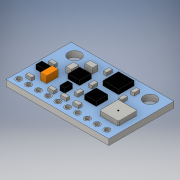
# Autodesk Inventor part: GY81
Saved by Autodesk Inventor 2016 (Build 200138000, 138)
## iProperties
Created: 2015-11-27
Part Number: GY81
Material: Generic
Document SubType Name: Modeling
Designer: Spooner
Density: 1 g/cm^3
Appearance: Default
Author: Spooner
Autodesk Inventor part; units mm, degrees
ref_plane "YZ Plane" through (0, 0, 0) normal (1, 0, 0) x (0, 1, 0)
ref_plane "XZ Plane" through (0, 0, 0) normal (0, 1, 0) x (-1, 0, 0)
ref_plane "XY Plane" through (0, 0, 0) normal (0, 0, 1) x (1, 0, 0)
sketch "Sketch1" plane through (0, 0, 0) normal (0, 1, 0) x (-1, 0, 0)
  line L0 (0, 0) -> (-26.67, 0)
  line L1 (-26.67, 0) -> (-26.67, -16.891)
  line L2 (-26.67, -16.891) -> (0, -16.891)
  line L3 (0, -16.891) -> (0, 0)
  circle A0 centre (-3.5369, -14.2431) radius 1.632
  circle A1 centre (-23.133, -14.2431) radius 1.632
  dimension "d0" = 16.891
  dimension "d1" = 26.67
  dimension "d2" = 3.2639
  dimension "d3" = 1.016
  dimension "d4" = 1.905
  dimension "d5" = 1.905
  constraints: 8 end point, 2 centre point, 2 parallel, 1 equal radius, 1 horizontal, 1 horizontal alignment, 1 perpendicular
  measures "d0" distance of L2.end L0.start
  measures "d1" distance of L1.end L2.end
  measures "d2" diameter of A0
  measures "d3" distance edge to line of A0 L2
  measures "d4" distance edge to line of A0 L3
  measures "d5" distance edge to line of A1 L1
extrude "Board" add sketch "Sketch1" along normal blind 1.524
sketch "Sketch2" plane through (0, 1.524, 0) normal (0, 1, 0) x (1, 0, 0)
  line L0 (20.1803, 4.0513) -> (25.0698, 4.0513)
  line L1 (25.0698, 4.0513) -> (25.0698, 8.9408)
  line L2 (25.0698, 8.9408) -> (20.1803, 8.9408)
  line L3 (20.1803, 8.9408) -> (20.1803, 4.0513)
  line L4 (26.67, 0) -> (26.67, 16.891) projected
  line L5 (26.67, 16.891) -> (0, 16.891) projected
  point P0 (0, 0)
  dimension "d8" = 4.8895
  dimension "d9" = 1.6002
  dimension "d10" = 7.9502
  constraints: 8 end point, 2 parallel, 2 perpendicular, 1 horizontal
  measures "d8" distance of L0.start L0.end
  measures "d9" distance between parallel lines of L4 L1
  measures "d10" distance between parallel lines of L2 L5
extrude "BMP085 Barometer" add sketch "Sketch2" along normal blind 1.1176
fillet "BMP085 Barometer Fillets" radius 0.254 4 edges at (25.0698, 2.0828, -4.0513) (20.1803, 2.0828, -4.0513) (20.1803, 2.0828, -8.9408) (25.0698, 2.0828, -8.9408)
sketch "Sketch3" plane through (0, 2.6416, 0) normal (0, 1, 0) x (1, 0, 0)
  circle A0 centre (22.6251, 6.4961) radius 0.1905
  line L0 (24.8158, 8.9408) -> (20.4343, 8.9408) projected
  line L1 (20.1803, 8.6868) -> (20.1803, 4.3053) projected
  point P0 (0, 0)
  point P1 (22.6251, 8.9408)
  point P2 (20.1803, 6.4961)
  dimension "d14" = 0.381
  constraints: 2 midpoint, 1 centre point, 1 horizontal alignment, 1 vertical alignment
  measures "d14" diameter of A0
extrude "BMP085 Barometer Hole" cut sketch "Sketch3" against normal blind 0.0254
sketch "Sketch4" plane through (0, 1.524, 0) normal (0, 1, 0) x (1, 0, 0)
  line L0 (13.97, 15.24) -> (18.034, 15.24)
  line L1 (18.034, 15.24) -> (18.034, 11.176)
  line L2 (18.034, 11.176) -> (13.97, 11.176)
  line L3 (13.97, 11.176) -> (13.97, 15.24)
  line L4 (14.7193, 8.6868) -> (17.7673, 8.6868)
  line L5 (17.7673, 8.6868) -> (17.7673, 5.6388)
  line L6 (17.7673, 5.6388) -> (14.7193, 5.6388)
  line L7 (14.7193, 5.6388) -> (14.7193, 8.6868)
  line L8 (7.874, 11.2141) -> (10.922, 11.2141)
  line L9 (10.922, 11.2141) -> (10.922, 8.1661)
  line L10 (10.922, 8.1661) -> (7.874, 8.1661)
  line L11 (7.874, 8.1661) -> (7.874, 11.2141)
  line L12 (9.4361, 6.5532) -> (10.7061, 6.5532)
  line L13 (10.7061, 6.5532) -> (10.7061, 4.5212)
  line L14 (10.7061, 4.5212) -> (9.4361, 4.5212)
  line L15 (9.4361, 4.5212) -> (9.4361, 6.5532)
  line L16 (1.6129, 7.6581) -> (4.1529, 7.6581)
  line L17 (4.1529, 7.6581) -> (4.1529, 6.1341)
  line L18 (4.1529, 6.1341) -> (1.6129, 6.1341)
  line L19 (1.6129, 6.1341) -> (1.6129, 7.6581)
  line L20 (26.67, 16.891) -> (0, 16.891) projected
  line L21 (26.67, 0) -> (26.67, 16.891) projected
  line L22 (20.1803, 4.3053) -> (20.1803, 8.6868) projected
  line L23 (0, 16.891) -> (0, 0) projected
  dimension "d17" = 4.064
  dimension "d18" = 3.048
  dimension "d19" = 1.27
  dimension "d20" = 2.032
  dimension "d21" = 1.524
  dimension "d22" = 2.54
  dimension "d23" = 1.651
  dimension "d24" = 8.636
  dimension "d25" = 2.413
  dimension "d26" = 2.4892
  dimension "d27" = 3.048
  dimension "d28" = 5.6769
  dimension "d29" = 4.0132
  dimension "d30" = 1.6129
  dimension "d31" = 1.6129
  dimension "d32" = 9.2329
  constraints: 40 end point, 10 parallel, 5 horizontal, 5 perpendicular, 4 equal length
  measures "d17" distance of L0.start L0.end
  measures "d18" distance of L4.start L4.end
  measures "d19" distance of L12.start L12.end
  measures "d20" distance of L14.end L12.start
  measures "d21" distance of L18.end L16.start
  measures "d22" distance of L16.start L16.end
  measures "d23" distance between parallel lines of L20 L0
  measures "d24" distance between parallel lines of L21 L1
  measures "d25" distance between parallel lines of L22 L5
  measures "d26" distance between parallel lines of L2 L4
  measures "d27" distance between parallel lines of L3 L9
  measures "d28" distance between parallel lines of L20 L8
  measures "d29" distance between parallel lines of L7 L13
  measures "d30" distance between parallel lines of L10 L12
  measures "d31" distance between parallel lines of L23 L19
  measures "d32" distance between parallel lines of L16 L20
extrude "Extrusion4" add sketch "Sketch4" along normal blind 1.1684
sketch "Sketch5" plane through (0, 1.524, 0) normal (0, 1, 0) x (1, 0, 0)
  line L0 (4.572, 7.366) -> (6.1849, 7.366)
  line L1 (6.1849, 7.366) -> (6.1849, 4.318)
  line L2 (6.1849, 4.318) -> (4.572, 4.318)
  line L3 (4.572, 4.318) -> (4.572, 7.366)
  line L4 (0, 0) -> (26.67, 0) projected
  line L5 (0, 16.891) -> (0, 0) projected
  dimension "d35" = 1.6129
  dimension "d36" = 3.048
  dimension "d74" = 4.318
  dimension "d75" = 4.572
  constraints: 8 end point, 2 parallel, 1 horizontal, 1 perpendicular
  measures "d35" distance of L1.end L2.end
  measures "d36" distance of L2.end L0.start
  measures "d74" distance between parallel lines of L4 L2
  measures "d75" distance between parallel lines of L5 L3
extrude "Extrusion5" add sketch "Sketch5" along normal blind 1.7399
sketch "Sketch6" plane through (0, 1.524, 0) normal (0, 1, 0) x (1, 0, 0)
  line L0 (8.0137, 13.843) -> (9.9949, 13.843)
  line L1 (9.9949, 13.843) -> (9.9949, 12.446)
  line L2 (9.9949, 12.446) -> (8.0137, 12.446)
  line L3 (8.0137, 12.446) -> (8.0137, 13.843)
  line L4 (0, 16.891) -> (0, 0) projected
  line L5 (6.2357, 11.2649) -> (7.6327, 11.2649)
  line L6 (7.6327, 11.2649) -> (7.6327, 9.2837)
  line L7 (7.6327, 9.2837) -> (6.2357, 9.2837)
  line L8 (6.2357, 9.2837) -> (6.2357, 11.2649)
  line L9 (26.67, 16.891) -> (0, 16.891) projected
  dimension "d39" = 1.9812
  dimension "d41" = 8.0137
  dimension "d42" = 1.397
  dimension "d43" = 6.2357
  dimension "d44" = 3.048
  dimension "d45" = 5.6261
  constraints: 16 end point, 4 parallel, 4 perpendicular, 2 horizontal
  measures "d39" distance of L0.start L0.end
  measures "d41" distance between parallel lines of L4 L3
  measures "d42" distance of L5.start L5.end
  measures "d43" distance between parallel lines of L4 L8
  measures "d44" distance between parallel lines of L0 L9
  measures "d45" distance between parallel lines of L5 L9
extrude "Extrusion6" add sketch "Sketch6" along normal blind 1.397
sketch "Sketch7" plane through (0, 1.524, 0) normal (0, 1, 0) x (1, 0, 0)
  line L0 (19.4691, 14.3256) -> (20.3708, 14.3256)
  line L1 (20.3708, 14.3256) -> (20.3708, 12.8397)
  line L2 (20.3708, 12.8397) -> (19.4691, 12.8397)
  line L3 (19.4691, 12.8397) -> (19.4691, 14.3256)
  line L4 (19.4691, 11.176) -> (20.3708, 11.176)
  line L5 (20.3708, 11.176) -> (20.3708, 9.6901)
  line L6 (20.3708, 9.6901) -> (19.4691, 9.6901)
  line L7 (19.4691, 9.6901) -> (19.4691, 11.176)
  line L8 (11.43, 15.3162) -> (12.2809, 15.3162)
  line L9 (12.2809, 15.3162) -> (12.2809, 13.8303)
  line L10 (12.2809, 13.8303) -> (11.43, 13.8303)
  line L11 (11.43, 13.8303) -> (11.43, 15.3162)
  line L12 (12.4206, 10.4902) -> (13.3223, 10.4902)
  line L13 (13.3223, 10.4902) -> (13.3223, 9.0043)
  line L14 (13.3223, 9.0043) -> (12.4206, 9.0043)
  line L15 (12.4206, 9.0043) -> (12.4206, 10.4902)
  line L16 (12.4206, 6.8072) -> (13.3223, 6.8072)
  line L17 (13.3223, 6.8072) -> (13.3223, 5.3213)
  line L18 (13.3223, 5.3213) -> (12.4206, 5.3213)
  line L19 (12.4206, 5.3213) -> (12.4206, 6.8072)
  line L20 (8.001, 3.7592) -> (9.4869, 3.7592)
  line L21 (9.4869, 3.7592) -> (9.4869, 2.8575)
  line L22 (9.4869, 2.8575) -> (8.001, 2.8575)
  line L23 (8.001, 2.8575) -> (8.001, 3.7592)
  line L24 (11.2395, 3.7592) -> (12.7254, 3.7592)
  line L25 (12.7254, 3.7592) -> (12.7254, 2.8575)
  line L26 (12.7254, 2.8575) -> (11.2395, 2.8575)
  line L27 (11.2395, 2.8575) -> (11.2395, 3.7592)
  line L28 (14.478, 3.7592) -> (15.9639, 3.7592)
  line L29 (15.9639, 3.7592) -> (15.9639, 2.8575)
  line L30 (15.9639, 2.8575) -> (14.478, 2.8575)
  line L31 (14.478, 2.8575) -> (14.478, 3.7592)
  line L32 (26.67, 16.891) -> (0, 16.891) projected
  line L33 (9.4361, 4.5212) -> (10.7061, 4.5212) projected
  line L34 (2.159, 9.6901) -> (3.6449, 9.6901)
  line L35 (3.6449, 9.6901) -> (3.6449, 8.8392)
  line L36 (3.6449, 8.8392) -> (2.159, 8.8392)
  line L37 (2.159, 8.8392) -> (2.159, 9.6901)
  line L38 (2.159, 3.81) -> (3.6449, 3.81)
  line L39 (3.6449, 3.81) -> (3.6449, 2.9591)
  line L40 (3.6449, 2.9591) -> (2.159, 2.9591)
  line L41 (2.159, 2.9591) -> (2.159, 3.81)
  line L42 (0, 16.891) -> (0, 0) projected
  line L43 (1.6129, 6.1341) -> (4.1529, 6.1341) projected
  line L44 (6.1849, 4.318) -> (6.1849, 7.366) projected
  line L45 (14.7193, 8.6868) -> (14.7193, 5.6388) projected
  line L46 (13.97, 15.24) -> (13.97, 11.176) projected
  line L47 (18.034, 11.176) -> (18.034, 15.24) projected
  point P0 (19.92, 12.8397)
  point P1 (19.92, 11.176)
  point P2 (12.8714, 9.0043)
  point P3 (12.8714, 6.8072)
  point P4 (2.159, 9.2647)
  point P5 (2.159, 3.3846)
  dimension "d48" = 0.8509
  dimension "d49" = 1.4859
  dimension "d50" = 1.5748
  dimension "d51" = 2.5654
  dimension "d52" = 1.6637
  dimension "d53" = 3.3401
  dimension "d54" = 2.1971
  dimension "d56" = 0.762
  dimension "d57" = 2.159
  dimension "d58" = 7.2009
  dimension "d59" = 2.3241
  dimension "d60" = 1.8161
  dimension "d61" = 1.7526
  dimension "d62" = 1.7526
  dimension "d63" = 0.9017
  dimension "d64" = 1.397
  dimension "d65" = 1.6891
  dimension "d66" = 1.4351
  constraints: 80 end point, 20 parallel, 14 equal length, 10 horizontal, 10 perpendicular, 7 point on line, 6 midpoint, 3 vertical alignment, 2 horizontal alignment
  measures "d48" distance of L8.start L8.end
  measures "d49" distance of L10.end L8.start
  measures "d50" distance between parallel lines of L32 L8
  measures "d51" distance between parallel lines of L0 L32
  measures "d52" distance of point (19.92, 12.84) point (19.92, 11.176)
  measures "d53" distance between parallel lines of L12 L10
  measures "d54" distance of point (12.871, 9.004) point (12.871, 6.807)
  measures "d56" distance between parallel lines of L33 L20
  measures "d57" distance from line of L42 point (2.159, 9.265)
  measures "d58" distance between parallel lines of L32 L34
  measures "d59" distance between parallel lines of L38 L43
  measures "d60" distance from line of L20.start L44
  measures "d61" distance between parallel lines of L27 L21
  measures "d62" distance between parallel lines of L31 L25
  measures "d63" distance of L29.end L28.end
  measures "d64" distance between parallel lines of L45 L17
  measures "d65" distance between parallel lines of L46 L9
  measures "d66" distance between parallel lines of L47 L3
extrude "Extrusion7" add sketch "Sketch7" along normal blind 0.762
sketch "Sketch8" plane through (0, 1.524, 0) normal (0, 1, 0) x (1, 0, 0)
  circle A0 centre (1.524, 1.778) radius 0.508
  line L0 (0, 0) -> (26.67, 0) projected
  line L1 (0, 16.891) -> (0, 0) projected
  dimension "d69" = 1.016
  dimension "d70" = 1.27
  dimension "d71" = 1.016
  constraints: 1 centre point
  measures "d69" diameter of A0
  measures "d70" distance edge to line of A0 L0
  measures "d71" distance edge to line of A0 L1
extrude "Extrusion8" cut sketch "Sketch8" against normal through all
sketch "Sketch9" plane through (0, 1.524, 0) normal (0, 1, 0) x (1, 0, 0)
  circle A0 centre (1.524, 1.778) radius 0.508 projected
  circle A1 centre (1.524, 1.778) radius 0.762
  point P0 (0, 0)
  dimension "d76" = 1.524
  constraints: 1 centre point, 1 coincident
  measures "d76" diameter of A1
extrude "Extrusion9" add sketch "Sketch9" along normal blind 0.0254
pattern_linear "Rectangular Pattern1" count 10 spacing 2.54 along (1, 0, 0) of "Extrusion8", "Extrusion9"
sketch "Sketch10" plane through (0, 0, 0) normal (0, -1, 0) x (1, 0, 0)
  circle A0 centre (24.384, -1.778) radius 0.508 projected
  circle A1 centre (21.844, -1.778) radius 0.508 projected
  circle A2 centre (19.304, -1.778) radius 0.508 projected
  circle A3 centre (16.764, -1.778) radius 0.508 projected
  circle A4 centre (14.224, -1.778) radius 0.508 projected
  circle A5 centre (11.684, -1.778) radius 0.508 projected
  circle A6 centre (9.144, -1.778) radius 0.508 projected
  circle A7 centre (6.604, -1.778) radius 0.508 projected
  circle A8 centre (4.064, -1.778) radius 0.508 projected
  circle A9 centre (1.524, -1.778) radius 0.508 projected
  circle A10 centre (23.133, -14.2431) radius 1.632 projected
  circle A11 centre (3.5369, -14.2431) radius 1.632 projected
  line L0 (0, 0) -> (26.67, 0) projected
  line L1 (0, -16.891) -> (0, 0) projected
  line L2 (26.67, -16.891) -> (0, -16.891) projected
  line L3 (26.67, 0) -> (26.67, -16.891) projected
  line L4 (0.8808, -8.8589) -> (0.8808, -2.794) construction
  line L5 (0.8808, -2.794) -> (2.1672, -2.794) construction
  line L6 (2.1672, -2.794) -> (2.1672, -8.8589) construction
  line L7 (2.1672, -8.8589) -> (0.8808, -8.8589) construction
  line L8 (5.9608, -8.8589) -> (5.9608, -2.794) construction
  line L9 (5.9608, -2.794) -> (7.2472, -2.794) construction
  line L10 (7.2472, -2.794) -> (7.2472, -8.8589) construction
  line L11 (7.2472, -8.8589) -> (5.9608, -8.8589) construction
  line L12 (8.5008, -8.8589) -> (8.5008, -2.794) construction
  line L13 (8.5008, -2.794) -> (9.7872, -2.794) construction
  line L14 (9.7872, -2.794) -> (9.7872, -8.8589) construction
  line L15 (9.7872, -8.8589) -> (8.5008, -8.8589) construction
  line L16 (11.0408, -8.8589) -> (11.0408, -2.794) construction
  line L17 (11.0408, -2.794) -> (12.3272, -2.794) construction
  line L18 (12.3272, -2.794) -> (12.3272, -8.8589) construction
  line L19 (12.3272, -8.8589) -> (11.0408, -8.8589) construction
  line L20 (1.0074, -7.9146) -> (2.0841, -8.2181)
  spline S0 degree 2 poles (2.0841, -8.2181) (2.1624, -8.2393) (2.1624, -8.3302) knots 0 0 0 1 1 1
  spline S1 degree 2 poles (2.1624, -8.3302) (2.1624, -8.422) (2.087, -8.4452) knots 0 0 0 1 1 1
  line L21 (2.087, -8.4452) -> (1.0122, -8.7864)
  spline S2 degree 2 poles (1.0122, -8.7864) (0.9958, -8.7903) (0.9794, -8.7903) knots 0 0 0 1 1 1
  spline S3 degree 2 poles (0.9794, -8.7903) (0.9417, -8.7903) (0.8904, -8.7342) (0.8904, -8.6965) knots 0 0 0 1 2 2 2
  spline S4 degree 2 poles (0.8904, -8.6965) (0.8904, -8.6327) (0.9774, -8.6115) knots 0 0 0 1 1 1
  line L22 (0.9774, -8.6115) -> (1.8618, -8.3321)
  line L23 (1.8618, -8.3321) -> (0.9523, -8.0886)
  spline S5 degree 2 poles (0.9523, -8.0886) (0.8904, -8.0721) (0.8904, -8.0074) knots 0 0 0 1 1 1
  spline S6 degree 2 poles (0.8904, -8.0074) (0.8904, -7.9707) (0.9426, -7.9107) (0.9823, -7.9107) knots 0 0 0 1 2 2 2
  spline S7 degree 2 poles (0.9823, -7.9107) (0.9958, -7.9107) (1.0074, -7.9146) knots 0 0 0 1 1 1
  spline S8 degree 2 poles (1.9652, -6.8166) (2.0793, -6.9094) (2.1672, -7.0863) (2.1672, -7.211) knots 0 0 0 1 2 2 2
  spline S9 degree 2 poles (2.1672, -7.211) (2.1672, -7.4236) (1.9874, -7.558) knots 0 0 0 1 1 1
  spline S10 degree 2 poles (1.9874, -7.558) (1.8057, -7.6962) (1.5119, -7.6962) knots 0 0 0 1 1 1
  spline S11 degree 2 poles (1.5119, -7.6962) (1.1872, -7.6962) (1.0171, -7.5406) knots 0 0 0 1 1 1
  spline S12 degree 2 poles (1.0171, -7.5406) (0.8808, -7.4159) (0.8808, -7.2361) knots 0 0 0 1 1 1
  spline S13 degree 2 poles (0.8808, -7.2361) (0.8808, -7.096) (0.9223, -7.0148) knots 0 0 0 1 1 1
  spline S14 degree 2 poles (0.9223, -7.0148) (0.9687, -6.9249) (1.0838, -6.8621) knots 0 0 0 1 1 1
  spline S15 degree 2 poles (1.0838, -6.8621) (1.1079, -6.8485) (1.1301, -6.8485) knots 0 0 0 1 1 1
  spline S16 degree 2 poles (1.1301, -6.8485) (1.1688, -6.8485) (1.222, -6.9065) (1.222, -6.9423) knots 0 0 0 1 2 2 2
  spline S17 degree 2 poles (1.222, -6.9423) (1.222, -6.9925) (1.1678, -7.0215) knots 0 0 0 1 1 1
  spline S18 degree 2 poles (1.1678, -7.0215) (1.1118, -7.0544) (1.0876, -7.1105) knots 0 0 0 1 1 1
  spline S19 degree 2 poles (1.0876, -7.1105) (1.0673, -7.153) (1.0673, -7.2371) knots 0 0 0 1 1 1
  spline S20 degree 2 poles (1.0673, -7.2371) (1.0673, -7.3463) (1.1649, -7.4217) knots 0 0 0 1 1 1
  spline S21 degree 2 poles (1.1649, -7.4217) (1.2829, -7.5145) (1.5119, -7.5145) knots 0 0 0 1 1 1
  spline S22 degree 2 poles (1.5119, -7.5145) (1.7226, -7.5145) (1.9807, -7.3395) (1.9807, -7.2081) knots 0 0 0 1 2 2 2
  spline S23 degree 2 poles (1.9807, -7.2081) (1.9807, -7.066) (1.8454, -6.9587) knots 0 0 0 1 1 1
  spline S24 degree 2 poles (1.8454, -6.9587) (1.8125, -6.9316) (1.8125, -6.8901) knots 0 0 0 1 1 1
  spline S25 degree 2 poles (1.8125, -6.8901) (1.8125, -6.8543) (1.8695, -6.7944) (1.9072, -6.7944) knots 0 0 0 1 2 2 2
  spline S26 degree 2 poles (1.9072, -6.7944) (1.9382, -6.7944) (1.9652, -6.8166) knots 0 0 0 1 1 1
  spline S27 degree 2 poles (1.9652, -5.6887) (2.0793, -5.7815) (2.1672, -5.9584) (2.1672, -6.083) knots 0 0 0 1 2 2 2
  spline S28 degree 2 poles (2.1672, -6.083) (2.1672, -6.2957) (1.9874, -6.43) knots 0 0 0 1 1 1
  spline S29 degree 2 poles (1.9874, -6.43) (1.8057, -6.5682) (1.5119, -6.5682) knots 0 0 0 1 1 1
  spline S30 degree 2 poles (1.5119, -6.5682) (1.1872, -6.5682) (1.0171, -6.4126) knots 0 0 0 1 1 1
  spline S31 degree 2 poles (1.0171, -6.4126) (0.8808, -6.288) (0.8808, -6.1082) knots 0 0 0 1 1 1
  spline S32 degree 2 poles (0.8808, -6.1082) (0.8808, -5.968) (0.9223, -5.8868) knots 0 0 0 1 1 1
  spline S33 degree 2 poles (0.9223, -5.8868) (0.9687, -5.797) (1.0838, -5.7341) knots 0 0 0 1 1 1
  spline S34 degree 2 poles (1.0838, -5.7341) (1.1079, -5.7206) (1.1301, -5.7206) knots 0 0 0 1 1 1
  spline S35 degree 2 poles (1.1301, -5.7206) (1.1688, -5.7206) (1.222, -5.7786) (1.222, -5.8144) knots 0 0 0 1 2 2 2
  spline S36 degree 2 poles (1.222, -5.8144) (1.222, -5.8646) (1.1678, -5.8936) knots 0 0 0 1 1 1
  spline S37 degree 2 poles (1.1678, -5.8936) (1.1118, -5.9265) (1.0876, -5.9825) knots 0 0 0 1 1 1
  spline S38 degree 2 poles (1.0876, -5.9825) (1.0673, -6.0251) (1.0673, -6.1091) knots 0 0 0 1 1 1
  spline S39 degree 2 poles (1.0673, -6.1091) (1.0673, -6.2184) (1.1649, -6.2937) knots 0 0 0 1 1 1
  spline S40 degree 2 poles (1.1649, -6.2937) (1.2829, -6.3865) (1.5119, -6.3865) knots 0 0 0 1 1 1
  spline S41 degree 2 poles (1.5119, -6.3865) (1.7226, -6.3865) (1.9807, -6.2116) (1.9807, -6.0801) knots 0 0 0 1 2 2 2
  spline S42 degree 2 poles (1.9807, -6.0801) (1.9807, -5.9381) (1.8454, -5.8308) knots 0 0 0 1 1 1
  spline S43 degree 2 poles (1.8454, -5.8308) (1.8125, -5.8037) (1.8125, -5.7622) knots 0 0 0 1 1 1
  spline S44 degree 2 poles (1.8125, -5.7622) (1.8125, -5.7264) (1.8695, -5.6665) (1.9072, -5.6665) knots 0 0 0 1 2 2 2
  spline S45 degree 2 poles (1.9072, -5.6665) (1.9382, -5.6665) (1.9652, -5.6887) knots 0 0 0 1 1 1
  line L24 (2.1421, -4.6371) -> (2.1421, -5.3901)
  spline S46 degree 2 poles (2.1421, -5.3901) (2.1421, -5.4838) (2.0503, -5.4838) knots 0 0 0 1 1 1
  spline S47 degree 2 poles (2.0503, -5.4838) (1.9613, -5.4838) (1.9613, -5.3901) knots 0 0 0 1 1 1
  line L25 (1.9613, -5.3901) -> (1.9613, -4.6371)
  spline S48 degree 2 poles (1.9613, -4.6371) (1.9613, -4.5444) (2.0503, -4.5444) knots 0 0 0 1 1 1
  spline S49 degree 2 poles (2.0503, -4.5444) (2.1421, -4.5444) (2.1421, -4.6371) knots 0 0 0 1 1 1
  spline S50 degree 2 poles (2.0628, -4.1964) (2.1585, -4.1964) (2.1585, -4.2882) knots 0 0 0 1 1 1
  spline S51 degree 2 poles (2.1585, -4.2882) (2.1585, -4.3801) (2.0628, -4.3801) knots 0 0 0 1 1 1
  line L26 (2.0628, -4.3801) -> (0.9852, -4.3801)
  spline S52 degree 2 poles (0.9852, -4.3801) (0.8924, -4.3801) (0.8924, -4.2882) knots 0 0 0 1 1 1
  spline S53 degree 2 poles (0.8924, -4.2882) (0.8924, -4.1964) (0.9852, -4.1964) knots 0 0 0 1 1 1
  line L27 (0.9852, -4.1964) -> (2.0628, -4.1964)
  spline S54 degree 2 poles (2.0667, -2.9419) (2.1604, -2.9419) (2.1604, -3.0202) knots 0 0 0 1 1 1
  spline S55 degree 2 poles (2.1604, -3.0202) (2.1604, -3.0753) (2.1092, -3.111) knots 0 0 0 1 1 1
  line L28 (2.1092, -3.111) -> (1.2278, -3.6861)
  line L29 (1.2278, -3.6861) -> (2.0648, -3.6861)
  spline S56 degree 2 poles (2.0648, -3.6861) (2.1604, -3.6861) (2.1604, -3.7779) knots 0 0 0 1 1 1
  spline S57 degree 2 poles (2.1604, -3.7779) (2.1604, -3.8697) (2.0648, -3.8697) knots 0 0 0 1 1 1
  line L30 (2.0648, -3.8697) -> (0.9774, -3.8697)
  spline S58 degree 2 poles (0.9774, -3.8697) (0.8885, -3.8697) (0.8885, -3.7847) knots 0 0 0 1 1 1
  spline S59 degree 2 poles (0.8885, -3.7847) (0.8885, -3.7286) (0.9446, -3.689) knots 0 0 0 1 1 1
  line L31 (0.9446, -3.689) -> (1.8028, -3.1255)
  line L32 (1.8028, -3.1255) -> (0.9832, -3.1255)
  spline S60 degree 2 poles (0.9832, -3.1255) (0.8885, -3.1255) (0.8885, -3.0337) knots 0 0 0 1 1 1
  spline S61 degree 2 poles (0.8885, -3.0337) (0.8885, -2.9419) (0.9832, -2.9419) knots 0 0 0 1 1 1
  line L33 (0.9832, -2.9419) -> (2.0667, -2.9419)
  spline S62 degree 2 poles (6.7765, -5.2741) (7.0326, -5.2741) (7.1583, -5.4152) knots 0 0 0 1 1 1
  spline S63 degree 2 poles (7.1583, -5.4152) (7.2472, -5.5147) (7.2472, -5.6472) knots 0 0 0 1 1 1
  spline S64 degree 2 poles (7.2472, -5.6472) (7.2472, -5.8723) (7.0143, -6.0231) knots 0 0 0 1 1 1
  spline S65 degree 2 poles (7.0143, -6.0231) (6.8548, -6.1536) (6.6132, -6.1536) knots 0 0 0 1 1 1
  spline S66 degree 2 poles (6.6132, -6.1536) (6.3184, -6.1536) (6.1425, -6.0173) knots 0 0 0 1 1 1
  spline S67 degree 2 poles (6.1425, -6.0173) (5.9608, -5.8791) (5.9608, -5.6674) knots 0 0 0 1 1 1
  spline S68 degree 2 poles (5.9608, -5.6674) (5.9608, -5.5196) (6.0381, -5.421) knots 0 0 0 1 1 1
  spline S69 degree 2 poles (6.0381, -5.421) (6.0603, -5.3756) (6.1551, -5.3127) knots 0 0 0 1 1 1
  spline S70 degree 2 poles (6.1551, -5.3127) (6.1802, -5.2953) (6.2101, -5.2953) knots 0 0 0 1 1 1
  spline S71 degree 2 poles (6.2101, -5.2953) (6.2469, -5.2953) (6.2981, -5.3514) (6.2981, -5.3872) knots 0 0 0 1 2 2 2
  spline S72 degree 2 poles (6.2981, -5.3872) (6.2981, -5.4345) (6.244, -5.4683) knots 0 0 0 1 1 1
  spline S73 degree 2 poles (6.244, -5.4683) (6.1956, -5.508) (6.1802, -5.5321) knots 0 0 0 1 1 1
  spline S74 degree 2 poles (6.1802, -5.5321) (6.1473, -5.5814) (6.1473, -5.6674) knots 0 0 0 1 1 1
  spline S75 degree 2 poles (6.1473, -5.6674) (6.1473, -5.8028) (6.4015, -5.97) (6.6132, -5.97) knots 0 0 0 1 2 2 2
  spline S76 degree 2 poles (6.6132, -5.97) (6.7852, -5.97) (6.9167, -5.8849) knots 0 0 0 1 1 1
  spline S77 degree 2 poles (6.9167, -5.8849) (7.0607, -5.7921) (7.0607, -5.6472) knots 0 0 0 1 1 1
  spline S78 degree 2 poles (7.0607, -5.6472) (7.0607, -5.5244) (6.935, -5.4838) knots 0 0 0 1 1 1
  spline S79 degree 2 poles (6.935, -5.4838) (6.8741, -5.4625) (6.7524, -5.4625) knots 0 0 0 1 1 1
  line L34 (6.7524, -5.4625) -> (6.7524, -5.6085)
  spline S80 degree 2 poles (6.7524, -5.6085) (6.7524, -5.7022) (6.6586, -5.7022) knots 0 0 0 1 1 1
  spline S81 degree 2 poles (6.6586, -5.7022) (6.5658, -5.7022) (6.5658, -5.6085) knots 0 0 0 1 1 1
  line L35 (6.5658, -5.6085) -> (6.5658, -5.2741)
  line L36 (6.5658, -5.2741) -> (6.7765, -5.2741)
  spline S82 degree 2 poles (7.1467, -4.0292) (7.2404, -4.0292) (7.2404, -4.1075) knots 0 0 0 1 1 1
  spline S83 degree 2 poles (7.2404, -4.1075) (7.2404, -4.1626) (7.1892, -4.1983) knots 0 0 0 1 1 1
  line L37 (7.1892, -4.1983) -> (6.3078, -4.7734)
  line L38 (6.3078, -4.7734) -> (7.1448, -4.7734)
  spline S84 degree 2 poles (7.1448, -4.7734) (7.2404, -4.7734) (7.2404, -4.8652) knots 0 0 0 1 1 1
  spline S85 degree 2 poles (7.2404, -4.8652) (7.2404, -4.9571) (7.1448, -4.9571) knots 0 0 0 1 1 1
  line L39 (7.1448, -4.9571) -> (6.0574, -4.9571)
  spline S86 degree 2 poles (6.0574, -4.9571) (5.9685, -4.9571) (5.9685, -4.872) knots 0 0 0 1 1 1
  spline S87 degree 2 poles (5.9685, -4.872) (5.9685, -4.8159) (6.0246, -4.7763) knots 0 0 0 1 1 1
  line L40 (6.0246, -4.7763) -> (6.8828, -4.2128)
  line L41 (6.8828, -4.2128) -> (6.0632, -4.2128)
  spline S88 degree 2 poles (6.0632, -4.2128) (5.9685, -4.2128) (5.9685, -4.121) knots 0 0 0 1 1 1
  spline S89 degree 2 poles (5.9685, -4.121) (5.9685, -4.0292) (6.0632, -4.0292) knots 0 0 0 1 1 1
  line L42 (6.0632, -4.0292) -> (7.1467, -4.0292)
  spline S90 degree 2 poles (6.56, -2.9071) (6.8993, -2.9071) (7.0771, -3.0869) knots 0 0 0 1 1 1
  spline S91 degree 2 poles (7.0771, -3.0869) (7.2221, -3.2318) (7.2221, -3.4425) knots 0 0 0 1 1 1
  line L43 (7.2221, -3.4425) -> (7.2221, -3.7798)
  line L44 (7.2221, -3.7798) -> (5.9724, -3.7798)
  line L45 (5.9724, -3.7798) -> (5.9724, -3.4435)
  spline S92 degree 2 poles (5.9724, -3.4435) (5.9724, -3.2357) (6.1096, -3.0849) knots 0 0 0 1 1 1
  spline S93 degree 2 poles (6.1096, -3.0849) (6.273, -2.9071) (6.56, -2.9071) knots 0 0 0 1 1 1
  spline S94 degree 2 poles (6.56, -3.0888) (6.3638, -3.0888) (6.2546, -3.2067) knots 0 0 0 1 1 1
  spline S95 degree 2 poles (6.2546, -3.2067) (6.1609, -3.3082) (6.1609, -3.4445) knots 0 0 0 1 1 1
  line L46 (6.1609, -3.4445) -> (6.1609, -3.5981)
  line L47 (6.1609, -3.5981) -> (7.0355, -3.5981)
  line L48 (7.0355, -3.5981) -> (7.0355, -3.4425)
  spline S96 degree 2 poles (7.0355, -3.4425) (7.0355, -3.3034) (6.9505, -3.2106) knots 0 0 0 1 1 1
  spline S97 degree 2 poles (6.9505, -3.2106) (6.8046, -3.0888) (6.56, -3.0888) knots 0 0 0 1 1 1
  spline S98 degree 2 poles (9.4301, -5.0643) (9.7964, -5.0643) (9.7964, -5.5167) knots 0 0 0 1 1 1
  spline S99 degree 2 poles (9.7964, -5.5167) (9.7964, -5.7883) (9.5248, -5.9352) knots 0 0 0 1 1 1
  spline S100 degree 2 poles (9.5248, -5.9352) (9.5074, -5.9458) (9.4803, -5.9458) knots 0 0 0 1 1 1
  spline S101 degree 2 poles (9.4803, -5.9458) (9.4398, -5.9458) (9.3769, -5.8859) (9.3769, -5.8472) knots 0 0 0 1 2 2 2
  spline S102 degree 2 poles (9.3769, -5.8472) (9.3769, -5.8008) (9.4195, -5.7825) knots 0 0 0 1 1 1
  spline S103 degree 2 poles (9.4195, -5.7825) (9.6099, -5.6964) (9.6099, -5.5167) knots 0 0 0 1 1 1
  spline S104 degree 2 poles (9.6099, -5.5167) (9.6099, -5.2518) (9.432, -5.2518) knots 0 0 0 1 1 1
  spline S105 degree 2 poles (9.432, -5.2518) (9.3441, -5.2518) (9.2745, -5.4181) knots 0 0 0 1 1 1
  spline S106 degree 2 poles (9.2745, -5.4181) (9.1401, -5.739) (9.1372, -5.7457) knots 0 0 0 1 1 1
  spline S107 degree 2 poles (9.1372, -5.7457) (9.0242, -5.9352) (8.8376, -5.9352) knots 0 0 0 1 1 1
  spline S108 degree 2 poles (8.8376, -5.9352) (8.6636, -5.9352) (8.5738, -5.8076) knots 0 0 0 1 1 1
  spline S109 degree 2 poles (8.5738, -5.8076) (8.5032, -5.7061) (8.4974, -5.5428) knots 0 0 0 1 1 1
  spline S110 degree 2 poles (8.4974, -5.5428) (8.4916, -5.392) (8.5699, -5.2702) knots 0 0 0 1 1 1
  spline S111 degree 2 poles (8.5699, -5.2702) (8.6337, -5.1581) (8.7651, -5.1165) knots 0 0 0 1 1 1
  spline S112 degree 2 poles (8.7651, -5.1165) (8.7864, -5.1107) (8.8009, -5.1107) knots 0 0 0 1 1 1
  spline S113 degree 2 poles (8.8009, -5.1107) (8.8395, -5.1107) (8.8869, -5.1678) (8.8869, -5.2045) knots 0 0 0 1 2 2 2
  spline S114 degree 2 poles (8.8869, -5.2045) (8.8869, -5.2721) (8.8347, -5.2886) knots 0 0 0 1 1 1
  spline S115 degree 2 poles (8.8347, -5.2886) (8.7555, -5.3137) (8.6762, -5.4519) (8.6801, -5.536) knots 0 0 0 1 2 2 2
  spline S116 degree 2 poles (8.6801, -5.536) (8.6888, -5.7535) (8.8337, -5.7535) knots 0 0 0 1 1 1
  spline S117 degree 2 poles (8.8337, -5.7535) (8.9101, -5.7535) (8.9633, -5.6771) knots 0 0 0 1 1 1
  spline S118 degree 2 poles (8.9633, -5.6771) (9.0039, -5.6201) (9.0531, -5.4838) knots 0 0 0 1 1 1
  spline S119 degree 2 poles (9.0531, -5.4838) (9.1276, -5.277) (9.1769, -5.2055) knots 0 0 0 1 1 1
  spline S120 degree 2 poles (9.1769, -5.2055) (9.2745, -5.0643) (9.4301, -5.0643) knots 0 0 0 1 1 1
  spline S121 degree 2 poles (9.5944, -3.9886) (9.7084, -4.0814) (9.7964, -4.2583) (9.7964, -4.3829) knots 0 0 0 1 2 2 2
  spline S122 degree 2 poles (9.7964, -4.3829) (9.7964, -4.5956) (9.6166, -4.7299) knots 0 0 0 1 1 1
  spline S123 degree 2 poles (9.6166, -4.7299) (9.4349, -4.8681) (9.1411, -4.8681) knots 0 0 0 1 1 1
  spline S124 degree 2 poles (9.1411, -4.8681) (8.8164, -4.8681) (8.6462, -4.7125) knots 0 0 0 1 1 1
  spline S125 degree 2 poles (8.6462, -4.7125) (8.51, -4.5879) (8.51, -4.4081) knots 0 0 0 1 1 1
  spline S126 degree 2 poles (8.51, -4.4081) (8.51, -4.2679) (8.5515, -4.1867) knots 0 0 0 1 1 1
  spline S127 degree 2 poles (8.5515, -4.1867) (8.5979, -4.0969) (8.7129, -4.034) knots 0 0 0 1 1 1
  spline S128 degree 2 poles (8.7129, -4.034) (8.7371, -4.0205) (8.7593, -4.0205) knots 0 0 0 1 1 1
  spline S129 degree 2 poles (8.7593, -4.0205) (8.798, -4.0205) (8.8511, -4.0785) (8.8511, -4.1143) knots 0 0 0 1 2 2 2
  spline S130 degree 2 poles (8.8511, -4.1143) (8.8511, -4.1645) (8.797, -4.1935) knots 0 0 0 1 1 1
  spline S131 degree 2 poles (8.797, -4.1935) (8.741, -4.2264) (8.7168, -4.2824) knots 0 0 0 1 1 1
  spline S132 degree 2 poles (8.7168, -4.2824) (8.6965, -4.325) (8.6965, -4.409) knots 0 0 0 1 1 1
  spline S133 degree 2 poles (8.6965, -4.409) (8.6965, -4.5183) (8.7941, -4.5936) knots 0 0 0 1 1 1
  spline S134 degree 2 poles (8.7941, -4.5936) (8.912, -4.6864) (9.1411, -4.6864) knots 0 0 0 1 1 1
  spline S135 degree 2 poles (9.1411, -4.6864) (9.3518, -4.6864) (9.6099, -4.5115) (9.6099, -4.3801) knots 0 0 0 1 2 2 2
  spline S136 degree 2 poles (9.6099, -4.3801) (9.6099, -4.238) (9.4745, -4.1307) knots 0 0 0 1 1 1
  spline S137 degree 2 poles (9.4745, -4.1307) (9.4417, -4.1036) (9.4417, -4.0621) knots 0 0 0 1 1 1
  spline S138 degree 2 poles (9.4417, -4.0621) (9.4417, -4.0263) (9.4987, -3.9664) (9.5364, -3.9664) knots 0 0 0 1 2 2 2
  spline S139 degree 2 poles (9.5364, -3.9664) (9.5673, -3.9664) (9.5944, -3.9886) knots 0 0 0 1 1 1
  line L49 (9.7732, -2.9805) -> (9.7732, -3.7325)
  line L50 (9.7732, -3.7325) -> (8.6163, -3.7325)
  spline S140 degree 2 poles (8.6163, -3.7325) (8.5216, -3.7325) (8.5216, -3.6407) knots 0 0 0 1 1 1
  spline S141 degree 2 poles (8.5216, -3.6407) (8.5216, -3.5508) (8.6163, -3.5508) knots 0 0 0 1 1 1
  line L51 (8.6163, -3.5508) -> (9.5886, -3.5508)
  line L52 (9.5886, -3.5508) -> (9.5886, -2.9805)
  spline S142 degree 2 poles (9.5886, -2.9805) (9.5886, -2.8887) (9.6794, -2.8887) knots 0 0 0 1 1 1
  spline S143 degree 2 poles (9.6794, -2.8887) (9.7732, -2.8887) (9.7732, -2.9805) knots 0 0 0 1 1 1
  spline S144 degree 2 poles (11.9701, -5.1359) (12.3364, -5.1359) (12.3364, -5.5882) knots 0 0 0 1 1 1
  spline S145 degree 2 poles (12.3364, -5.5882) (12.3364, -5.8598) (12.0648, -6.0067) knots 0 0 0 1 1 1
  spline S146 degree 2 poles (12.0648, -6.0067) (12.0474, -6.0173) (12.0203, -6.0173) knots 0 0 0 1 1 1
  spline S147 degree 2 poles (12.0203, -6.0173) (11.9798, -6.0173) (11.9169, -5.9574) (11.9169, -5.9187) knots 0 0 0 1 2 2 2
  spline S148 degree 2 poles (11.9169, -5.9187) (11.9169, -5.8723) (11.9595, -5.854) knots 0 0 0 1 1 1
  spline S149 degree 2 poles (11.9595, -5.854) (12.1499, -5.768) (12.1499, -5.5882) knots 0 0 0 1 1 1
  spline S150 degree 2 poles (12.1499, -5.5882) (12.1499, -5.3234) (11.972, -5.3234) knots 0 0 0 1 1 1
  spline S151 degree 2 poles (11.972, -5.3234) (11.8841, -5.3234) (11.8145, -5.4896) knots 0 0 0 1 1 1
  spline S152 degree 2 poles (11.8145, -5.4896) (11.6801, -5.8105) (11.6772, -5.8173) knots 0 0 0 1 1 1
  spline S153 degree 2 poles (11.6772, -5.8173) (11.5642, -6.0067) (11.3776, -6.0067) knots 0 0 0 1 1 1
  spline S154 degree 2 poles (11.3776, -6.0067) (11.2036, -6.0067) (11.1138, -5.8791) knots 0 0 0 1 1 1
  spline S155 degree 2 poles (11.1138, -5.8791) (11.0432, -5.7776) (11.0374, -5.6143) knots 0 0 0 1 1 1
  spline S156 degree 2 poles (11.0374, -5.6143) (11.0316, -5.4635) (11.1099, -5.3417) knots 0 0 0 1 1 1
  spline S157 degree 2 poles (11.1099, -5.3417) (11.1737, -5.2296) (11.3051, -5.1881) knots 0 0 0 1 1 1
  spline S158 degree 2 poles (11.3051, -5.1881) (11.3264, -5.1823) (11.3409, -5.1823) knots 0 0 0 1 1 1
  spline S159 degree 2 poles (11.3409, -5.1823) (11.3795, -5.1823) (11.4269, -5.2393) (11.4269, -5.276) knots 0 0 0 1 2 2 2
  spline S160 degree 2 poles (11.4269, -5.276) (11.4269, -5.3437) (11.3747, -5.3601) knots 0 0 0 1 1 1
  spline S161 degree 2 poles (11.3747, -5.3601) (11.2955, -5.3852) (11.2162, -5.5234) (11.2201, -5.6075) knots 0 0 0 1 2 2 2
  spline S162 degree 2 poles (11.2201, -5.6075) (11.2288, -5.825) (11.3737, -5.825) knots 0 0 0 1 1 1
  spline S163 degree 2 poles (11.3737, -5.825) (11.4501, -5.825) (11.5033, -5.7486) knots 0 0 0 1 1 1
  spline S164 degree 2 poles (11.5033, -5.7486) (11.5439, -5.6916) (11.5931, -5.5553) knots 0 0 0 1 1 1
  spline S165 degree 2 poles (11.5931, -5.5553) (11.6676, -5.3485) (11.7169, -5.277) knots 0 0 0 1 1 1
  spline S166 degree 2 poles (11.7169, -5.277) (11.8145, -5.1359) (11.9701, -5.1359) knots 0 0 0 1 1 1
  spline S167 degree 2 poles (11.6492, -4.0572) (11.9885, -4.0572) (12.1663, -4.237) knots 0 0 0 1 1 1
  spline S168 degree 2 poles (12.1663, -4.237) (12.3113, -4.382) (12.3113, -4.5927) knots 0 0 0 1 1 1
  line L53 (12.3113, -4.5927) -> (12.3113, -4.93)
  line L54 (12.3113, -4.93) -> (11.0616, -4.93)
  line L55 (11.0616, -4.93) -> (11.0616, -4.5936)
  spline S169 degree 2 poles (11.0616, -4.5936) (11.0616, -4.3858) (11.1988, -4.2351) knots 0 0 0 1 1 1
  spline S170 degree 2 poles (11.1988, -4.2351) (11.3622, -4.0572) (11.6492, -4.0572) knots 0 0 0 1 1 1
  spline S171 degree 2 poles (11.6492, -4.2389) (11.453, -4.2389) (11.3438, -4.3569) knots 0 0 0 1 1 1
  spline S172 degree 2 poles (11.3438, -4.3569) (11.25, -4.4583) (11.25, -4.5946) knots 0 0 0 1 1 1
  line L56 (11.25, -4.5946) -> (11.25, -4.7483)
  line L57 (11.25, -4.7483) -> (12.1247, -4.7483)
  line L58 (12.1247, -4.7483) -> (12.1247, -4.5927)
  spline S173 degree 2 poles (12.1247, -4.5927) (12.1247, -4.4535) (12.0397, -4.3607) knots 0 0 0 1 1 1
  spline S174 degree 2 poles (12.0397, -4.3607) (11.8937, -4.2389) (11.6492, -4.2389) knots 0 0 0 1 1 1
  spline S175 degree 2 poles (12.205, -2.8549) (12.2243, -2.8481) (12.2407, -2.8481) knots 0 0 0 1 1 1
  spline S176 degree 2 poles (12.2407, -2.8481) (12.2803, -2.8481) (12.3296, -2.9071) (12.3296, -2.9428) knots 0 0 0 1 2 2 2
  spline S177 degree 2 poles (12.3296, -2.9428) (12.3296, -3.0057) (12.2716, -3.0279) knots 0 0 0 1 1 1
  line L59 (12.2716, -3.0279) -> (12.0996, -3.0946)
  line L60 (12.0996, -3.0946) -> (12.0996, -3.6561)
  line L61 (12.0996, -3.6561) -> (12.2707, -3.7219)
  spline S178 degree 2 poles (12.2707, -3.7219) (12.3296, -3.7441) (12.3296, -3.805) knots 0 0 0 1 1 1
  spline S179 degree 2 poles (12.3296, -3.805) (12.3296, -3.8436) (12.2794, -3.9007) (12.2407, -3.9007) knots 0 0 0 1 2 2 2
  spline S180 degree 2 poles (12.2407, -3.9007) (12.2233, -3.9007) (12.2079, -3.8949) knots 0 0 0 1 1 1
  line L62 (12.2079, -3.8949) -> (11.1196, -3.4889)
  spline S181 degree 2 poles (11.1196, -3.4889) (11.05, -3.4628) (11.05, -3.3836) knots 0 0 0 1 1 1
  spline S182 degree 2 poles (11.05, -3.3836) (11.05, -3.3024) (11.1109, -3.2802) knots 0 0 0 1 1 1
  line L63 (11.1109, -3.2802) -> (12.205, -2.8549)
  line L64 (11.9131, -3.1574) -> (11.3216, -3.3836)
  line L65 (11.3216, -3.3836) -> (11.9131, -3.5943)
  line L66 (11.9131, -3.5943) -> (11.9131, -3.1574)
  point P0 (7.0437, -1.778)
  point P1 (1.524, -2.794)
  point P2 (6.604, -2.794)
  point P3 (9.144, -2.794)
  point P4 (11.684, -2.794)
  dimension "d82" = 1.016
  constraints: 4 horizontal alignment, 4 midpoint, 4 vertical alignment, 8 other
  measures "d82" distance from line of A9.centre L5
extrude "Extrusion10" add sketch "Sketch10" along normal blind 0.0254 contours L20 S0 S1 L21 S2 S3 S4 L22 L23 S5 S6 S7 | S8 S9 S10 S11 S12 S13 S14 S15 S16 S17 S18 S19 S20 S21 S22 S23 S24 S25 S26 | S27 S28 S29 S30 S31 S32 S33 S34 S35 S36 S37 S38 S39 S40 S41 S42 S43 S44 S45 | L24 S46 S47 L25 S48 S49 | S50 S51 L26 S52 S53 L27 | S54 S55 L28 L29 S56 S57 L30 S58 S59 L31 L32 S60 S61 L33 | S62 S63 S64 S65 S66 S67 S68 S69 S70 S71 S72 S73 S74 S75 S76 S77 S78 S79 L34 S80 S81 L35 L36 | S82 S83 L37 L38 S84 S85 L39 S86 S87 L40 L41 S88 S89 L42 | S90 S91 L43 L44 L45 S92 S93 | S98 S99 S100 S101 S102 S103 S104 S105 S106 S107 S108 S109 S110 S111 S112 S113 S114 S115 S116 S117 S118 S119 S120 | S121 S122 S123 S124 S125 S126 S127 S128 S129 S130 S131 S132 S133 S134 S135 S136 S137 S138 S139 | L49 L50 S140 S141 L51 L52 S142 S143 | S144 S145 S146 S147 S148 S149 S150 S151 S152 S153 S154 S155 S156 S157 S158 S159 S160 S161 S162 S163 S164 S165 S166 | S167 S168 L53 L54 L55 S169 S170 | S175 S176 S177 L59 L60 L61 S178 S179 S180 L62 S181 S182 L63
equation "\"d5\" = d4"
equation "\"d62\" = d61"
body "Solid1"
